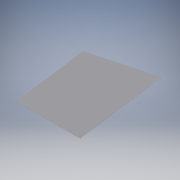
# Autodesk Inventor part: panelDflat.KR
Saved by Autodesk Inventor 2016 (Build 200138000, 138)
## iProperties
Created: 2015-02-13
Part Number: panelDflat.KR
Material: Generic
Document SubType Name: Modeling
Designer: Dave
Density: 1 g/cm^3
Appearance: Default
Author: Dave
Autodesk Inventor part; units mm, degrees
ref_plane "YZ Plane" through (0, 0, 0) normal (1, 0, 0) x (0, 1, 0)
ref_plane "XZ Plane" through (0, 0, 0) normal (0, 1, 0) x (-1, 0, 0)
ref_plane "XY Plane" through (0, 0, 0) normal (0, 0, 1) x (1, 0, 0)
sketch "Sketch1" plane through (0, 0, 0) normal (0, 1, 0) x (-1, 0, 0)
  line L0 (0, 0) -> (-12000, 0) construction
  line L1 (0, 0) -> (-11591.1099, -3105.8285) construction
  line L2 (0, 0) -> (12000, 0) construction
  line L3 (-6551.7777, 50) -> (-6315.5903, -1744.0211)
  line L4 (-5127.7716, -1425.7461) -> (-5322.0572, 50)
  line L5 (0, 0) -> (-5224.9144, -687.873) construction
  line L6 (0, 0) -> (5270, 0) construction
  line L7 (-5127.7716, -1425.7461) -> (-6315.5903, -1744.0211)
  line L8 (-5322.0572, 50) -> (-6551.7777, 50)
  dimension "d2" = 165
  dimension "d5" = 5270
  dimension "d6" = 172.5
  dimension "d7" = 50
  dimension "d8" = 50
  constraints: 18 end point, 3 horizontal, 3 parallel, 2 equal length, 1 midpoint, 1 perpendicular
  measures "d2" angle of L1 L2
  measures "d5" distance of L5.end L0.start
  measures "d6" angle of L5 L6
  measures "d7" distance between parallel lines of L1 L7
  measures "d8" distance between parallel lines of L8 L0
extrude "Extrusion1" add sketch "Sketch1" along normal blind 1
body "Solid1"
